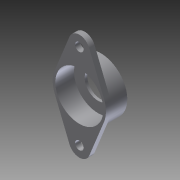
# Autodesk Inventor part: bearing block wheel mount
Saved by Autodesk Inventor 2012 (Build 160160000, 160)
## iProperties
Created: 2012-02-08
Part Number: bearing block wheel mount
Material: Default
Document SubType Name: Modeling
Designer: Antonella Wilby
Density: 1 g/cm^3
Author: Antonella Wilby
Autodesk Inventor part; units mm, degrees
ref_plane "YZ Plane" through (0, 0, 0) normal (1, 0, 0) x (0, 1, 0)
ref_plane "XZ Plane" through (0, 0, 0) normal (0, 1, 0) x (-1, 0, 0)
ref_plane "XY Plane" through (0, 0, 0) normal (0, 0, 1) x (1, 0, 0)
sketch "Sketch1" plane through (0, 0, 0) normal (0, 0, 1) x (1, 0, 0)
  circle A0 centre (0, 0) radius 14.2875 construction
  line L0 (-22.225, 0) -> (22.225, 0) projected
  line L1 (0, -44.45) -> (0, 44.45) projected
  arc A1 (5.8866, 27.7812) -> (-5.8866, 27.7812) centre (0, 25.4) ccw
  arc A2 (-5.8866, -27.7812) -> (5.8866, -27.7812) centre (0, -25.4) ccw
  line L2 (5.8866, -27.7812) -> (14.7165, -5.9531)
  line L3 (-5.8866, -27.7812) -> (-14.7165, -5.9531)
  line L4 (-5.8866, 27.7812) -> (-14.7165, 5.9531)
  line L5 (5.8866, 27.7812) -> (14.7165, 5.9531)
  arc A3 (-14.7165, 5.9531) -> (-14.7165, -5.9531) centre (0, 0) ccw
  arc A4 (14.7165, -5.9531) -> (14.7165, 5.9531) centre (0, 0) ccw
  circle A5 centre (0, 0) radius 7.9375
  dimension "d1" = 28.575
  dimension "d2" = 15.875
  dimension "d3" = 15.875
  dimension "d4" = 6.35
  dimension "d5" = 25.4
  dimension "d6" = 25.4
  dimension "d7" = 15.875
  constraints: 8 end point, 8 point on circle, 8 tangent, 6 centre point, 3 coincident, 2 point on line, 1 equal radius
  measures "d1" diameter of A0
  measures "d2" radius of A4
  measures "d3" radius of A3
  measures "d4" radius of A1
  measures "d5" distance from line of A1.centre L0
  measures "d6" distance from line of L0 A2.centre
  measures "d7" diameter of A5
extrude "Extrusion1" add sketch "Sketch1" against normal blind 12.7 contours A3 L4 A1 L1 A5 L0 | L0 A5 L1 A2 L3 A3 | L1 A1 L5 A4 L0 A5 | A5 L0 A4 L2 A2 L1
sketch "Sketch2" plane through (0, 0, -12.7) normal (0, 0, -1) x (-1, 0, 0)
  line L0 (-5.8866, -27.7812) -> (-14.7165, -5.9531) projected
  arc A0 (-5.8866, -27.7812) -> (5.8866, -27.7812) centre (0, -25.4) ccw projected
  line L1 (14.7165, -5.9531) -> (5.8866, -27.7812) projected
  arc A1 (14.7165, -5.9531) -> (14.7165, 5.9531) centre (0, 0) ccw projected
  line L2 (5.8866, 27.7812) -> (14.7165, 5.9531) projected
  arc A2 (5.8866, 27.7812) -> (-5.8866, 27.7812) centre (0, 25.4) ccw projected
  line L3 (-14.7165, 5.9531) -> (-5.8866, 27.7812) projected
  arc A3 (-14.7165, 5.9531) -> (-14.7165, -5.9531) centre (0, 0) ccw projected
  circle A4 centre (0, 0) radius 15.875
  constraints: 1 centre point, 1 coincident, 1 concentric
extrude "Extrusion2" cut sketch "Sketch2" against normal blind 9.525 contours L0 A4 L1 A0 | L3 A2 L2 A4
sketch "Sketch3" plane through (0, 0, 0) normal (0, 0, 1) x (1, 0, 0)
  circle A0 centre (0, 0) radius 7.9375 projected
  arc A1 (-14.7165, 5.9531) -> (-14.7165, -5.9531) centre (0, 0) ccw projected
  circle A2 centre (0, 0) radius 14.3129
  dimension "d12" = 28.6258
  constraints: 1 centre point, 1 coincident
  measures "d12" diameter of A2
extrude "Extrusion3" cut sketch "Sketch3" against normal blind 11.1125
sketch "Sketch4" plane through (0, 0, 0) normal (0, 0, 1) x (1, 0, 0)
  arc A0 (-5.8866, -27.7812) -> (5.8866, -27.7812) centre (0, -25.4) ccw projected
  arc A1 (5.8866, 27.7812) -> (-5.8866, 27.7812) centre (0, 25.4) ccw projected
  constraints: 2 coincident
hole "Hole1" at (0, 25.4, 0) at (0, -25.4, 0) direction (0, 0, -1) diameter 5.1054 end through all clearance for "Flat Head Machine Screw (82)" size "#10" standard "Ansi Unified Screw Threads"
body "Solid1"
